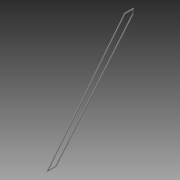
# Autodesk Inventor part: steel cable
Saved by Autodesk Inventor 2015 SP1 (Build 190203100, 203)
## iProperties
Created: 2015-01-27
Part Number: steel cable
Material: Generic
Document SubType Name: Modeling
Designer: Admin
Density: 1 g/cm^3
Appearance: Default
Author: Admin
Autodesk Inventor part; units mm, degrees
ref_plane "YZ Plane" through (0, 0, 0) normal (1, 0, 0) x (0, 1, 0)
ref_plane "XZ Plane" through (0, 0, 0) normal (0, 1, 0) x (-1, 0, 0)
ref_plane "XY Plane" through (0, 0, 0) normal (0, 0, 1) x (1, 0, 0)
sketch "Sketch1" plane through (0, 0, 0) normal (1, 0, 0) x (0, 1, 0)
  line L0 (295.5825, -234.2099) -> (295.5825, -259.6099)
  line L1 (295.5825, -259.6099) -> (282.8825, -259.6099)
  line L2 (282.8825, -259.6099) -> (0, -25.4)
  line L3 (0, -25.4) -> (0, 0)
  line L4 (0, 0) -> (295.5825, -234.2099)
  point P0 (0, 0)
  dimension "d0" = 0
  dimension "d1" = 0
  dimension "d2" = 25.4
  dimension "d3" = 0
  dimension "d4" = 25.4
  dimension "d5" = 12.7
  constraints: 10 end point, 1 perpendicular, 1 vertical
  measures "d0" distance of point (0, 0) L3.end
  measures "d1" distance of point (0, 0) L3.end
  measures "d2" distance of L2.end L3.end
  measures "d3" horizontal distance of L2.end L3.end
  measures "d4" distance of L0.start L0.end
  measures "d5" distance of L0.end L1.end
sketch "Sketch2" plane through (0, 0, 0) normal (0, 0, 1) x (1, 0, 0)
  circle A0 centre (0, 0) radius 1.5875
  dimension "d6" = 3.175
  constraints: 1 centre point, 1 coincident
  measures "d6" diameter of A0
sweep "Sweep1" add profiles "Sketch2" path "Sketch1" path curves L3 L2 L1 L0 L4
body "Solid1"
